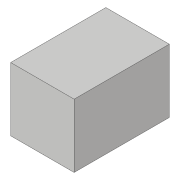
# Autodesk Inventor part: formingToolMain
Saved by Autodesk Inventor 2018 (Build 220112000, 112)
## iProperties
Created: 2020-04-02
Part Number: formingToolMain
Material: Generic
Document SubType Name: Modeling
Designer: Matt
Density: 1 g/cm^3
Appearance: Default
Author: Matt
Autodesk Inventor part; units mm, degrees
ref_plane "YZ Plane" through (0, 0, 0) normal (1, 0, 0) x (0, 1, 0)
ref_plane "XZ Plane" through (0, 0, 0) normal (0, 1, 0) x (-1, 0, 0)
ref_plane "XY Plane" through (0, 0, 0) normal (0, 0, 1) x (1, 0, 0)
sketch "Sketch1" plane through (0, 0, 0) normal (0, 1, 0) x (-1, 0, 0)
  line L0 (-50.8, 76.2) -> (50.8, 76.2)
  line L1 (50.8, 76.2) -> (50.8, -76.2)
  line L2 (50.8, -76.2) -> (-50.8, -76.2)
  line L3 (-50.8, -76.2) -> (-50.8, 76.2)
  line L4 (-50.8, 76.2) -> (50.8, -76.2) construction
  line L5 (50.8, 76.2) -> (-50.8, -76.2) construction
  point P0 (0, 0)
  dimension "d0" = 101.6
  dimension "d1" = 152.4
  constraints: 12 end point, 2 midpoint, 2 parallel, 1 horizontal, 1 perpendicular
  measures "d0" distance of L1.end L2.end
  measures "d1" distance of L0.end L1.end
extrude "Extrusion1" add sketch "Sketch1" along normal blind 101.6
body "Solid1"
